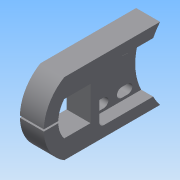
# Autodesk Inventor part: motormount2
Saved by Autodesk Inventor 2015 (Build 190159000, 159)
## iProperties
Created: 2015-12-05
Part Number: motormount2
Material: Generic
Document SubType Name: Modeling
Designer: JoshuaYuan
Density: 1 g/cm^3
Appearance: Default
Author: JoshuaYuan
Autodesk Inventor part; units mm, degrees
ref_plane "YZ Plane" through (0, 0, 0) normal (1, 0, 0) x (0, 1, 0)
ref_plane "XZ Plane" through (0, 0, 0) normal (0, 1, 0) x (-1, 0, 0)
ref_plane "XY Plane" through (0, 0, 0) normal (0, 0, 1) x (1, 0, 0)
sketch "Sketch1" plane through (0, 0, 0) normal (1, 0, 0) x (0, 1, 0)
  line L0 (57.5224, -43.6936) -> (57.5224, -57.6636)
  line L1 (57.5224, -57.6636) -> (39.4884, -57.6636)
  line L2 (39.4884, -57.6636) -> (39.4884, -43.6936)
  arc A0 (57.5224, -43.6936) -> (49.0054, -40.5737) centre (48.5054, -55.1236) ccw
  line L3 (67.5554, -43.7679) -> (67.5554, -94.5433)
  line L4 (29.4554, -43.7679) -> (29.4554, -94.5433)
  arc A1 (67.5554, -43.7679) -> (49.0054, -32.9515) centre (48.5054, -55.1236) ccw
  arc A2 (67.5554, -94.5433) -> (29.4554, -94.5433) centre (48.5054, -117.7186) ccw
  line L5 (60.5196, -70.9986) -> (60.5196, -67.8236)
  line L6 (55.5412, -67.8236) -> (55.5412, -70.9986)
  arc A3 (60.5196, -67.8236) -> (55.5412, -67.8236) centre (58.0304, -67.8236) ccw
  arc A4 (55.5412, -70.9986) -> (60.5196, -70.9986) centre (58.0304, -70.9986) ccw
  arc A5 (60.5196, -80.5236) -> (55.5412, -80.5236) centre (58.0304, -80.5236) ccw
  line L7 (60.5196, -83.6986) -> (60.5196, -80.5236)
  arc A6 (55.5412, -83.6986) -> (60.5196, -83.6986) centre (58.0304, -83.6986) ccw
  line L8 (55.5412, -80.5236) -> (55.5412, -83.6986)
  arc A7 (41.4696, -67.8236) -> (36.4912, -67.8236) centre (38.9804, -67.8236) ccw
  line L9 (41.4696, -70.9986) -> (41.4696, -67.8236)
  arc A8 (36.4912, -70.9986) -> (41.4696, -70.9986) centre (38.9804, -70.9986) ccw
  line L10 (36.4912, -67.8236) -> (36.4912, -70.9986)
  arc A9 (41.4696, -80.5236) -> (36.4912, -80.5236) centre (38.9804, -80.5236) ccw
  line L11 (41.4696, -83.6986) -> (41.4696, -80.5236)
  arc A10 (36.4912, -83.6986) -> (41.4696, -83.6986) centre (38.9804, -83.6986) ccw
  line L12 (36.4912, -80.5236) -> (36.4912, -83.6986)
  line L13 (48.5054, -117.7186) -> (48.5054, -32.9436) construction
  line L14 (57.5224, -50.6786) -> (39.4884, -50.6786) construction
  line L15 (48.0054, -40.5737) -> (48.0054, -32.9515)
  line L16 (49.0054, -32.9515) -> (49.0054, -40.5737)
  arc A11 (49.0054, -32.9515) -> (48.0054, -32.9515) centre (48.5054, -55.1236) ccw construction
  arc A12 (48.0054, -32.9515) -> (29.4554, -43.7679) centre (48.5054, -55.1236) ccw
  arc A13 (48.0054, -40.5737) -> (39.4884, -43.6936) centre (48.5054, -55.1236) ccw
  arc A14 (49.0054, -40.5737) -> (48.0054, -40.5737) centre (48.5054, -55.1236) ccw construction
  point P0 (0, 0)
  point P1 (48.5054, -40.5636)
  point P2 (48.5054, -50.6786)
  dimension "d0" = 13.97
  dimension "d1" = 18.034
  dimension "d2" = 2.54
  dimension "d4" = 30
  dimension "d8" = 4.9784
  dimension "d9" = 2.4892
  dimension "d17" = 3.175
  dimension "d20" = 12.7
  dimension "d23" = 19.05
  dimension "d26" = 38.1
  dimension "d30" = 10.16
  dimension "d31" = 7.62
  dimension "d32" = 67.04
  dimension "d33" = 1
  constraints: 34 end point, 32 point on circle, 15 centre point, 7 vertical, 3 midpoint, 3 parallel, 2 coincident, 2 perpendicular, 2 point on line, 1 concentric, 1 equal radius, 1 horizontal, 32 other
  measures "d0" distance of L0.start L0.end
  measures "d1" distance of L0.end L1.end
  measures "d2" distance from line of L1 A0.centre
  measures "d4" radius of A2
  measures "d8" distance between parallel lines of L6 L5
  measures "d9" radius of A4
  measures "d17" distance of L6.start L6.end
  measures "d20" distance of L6.start L8.start
  measures "d23" distance of L6.start L10.start
  measures "d26" distance between parallel lines of L4 L3
  measures "d30" distance from line of L1 A7.centre
  measures "d31" distance of point (48.505, -32.944) point (48.505, -40.564)
  measures "d32" distance of point (48.505, -50.679) A2.centre
  measures "d33" distance between parallel lines of L15 L16
extrude "Extrusion1" add sketch "Sketch1" along normal blind 12.7
sketch "Sketch2" plane through (12.7, 0, 0) normal (1, 0, 0) x (0, 0, -1)
  arc A0 (94.5433, 67.5554) -> (94.5433, 29.4554) centre (117.7186, 48.5054) ccw projected
  line L0 (90.8936, 61.9374) -> (64.8078, 61.9374)
  line L1 (62.3186, 59.4482) -> (62.3186, 37.5626)
  line L2 (64.8078, 35.0734) -> (90.8936, 35.0734)
  line L3 (87.7186, 48.5054) -> (62.3186, 48.5054) construction
  arc A1 (64.8078, 61.9374) -> (62.3186, 59.4482) centre (64.8078, 59.4482) ccw
  arc A2 (62.3186, 37.5626) -> (64.8078, 35.0734) centre (64.8078, 37.5626) ccw
  point P0 (0, 0)
  point P1 (62.3186, 61.9374)
  dimension "d37" = 25.4
  dimension "d38" = 28.575
  dimension "d39" = 2.4892
  constraints: 8 end point, 7 point on circle, 4 tangent, 3 perpendicular, 2 centre point, 2 point on line, 1 equal radius, 1 horizontal, 1 midpoint, 1 other
  measures "d37" distance of L3.start L3.end
  measures "d38" distance of L0.start point (62.319, 61.937)
  measures "d39" radius of A1
extrude "Extrusion2" cut sketch "Sketch2" against normal blind 6.35
body "Solid1"
